Storagebar (Autodesk Fusion 360 design; units mm, degrees)
Autodesk Fusion 360 part; units mm, degrees
sketch "Sketch1" plane through (0, 0, 0) normal (1, 0, 0) x (0, 1, 0)
  circle A0 centre (0, 0) radius 9
  dimension "d1" = 18
  constraint coincident A0.centre origin
  measures "d1" diameter of A0
extrude "Extrude1" add sketch "Sketch1" along normal blind 100 from surface at 5 makes body 1
sketch "Sketch2" plane through (0, 0, 0) normal (1, 0, 0) x (0, 1, 0)
  circle A0 centre (0, 0) radius 9.1
  circle A1 centre (0, 0) radius 12.6
  line L0 (0, 0) -> (-19.9239, 1.7431)
  line L1 (0, 0) -> (20, 0) construction
  line L2 (0, 0) -> (19.9239, 1.7431)
  line L3 (0, 0) -> (20, 0) construction
  circle A2 centre (0, -35) radius 10
  circle A3 centre (0, -35) radius 5
  line L4 (-21.2876, 35.0304) -> (-21.2876, -70)
  line L5 (-13.3685, 9.8483) -> (-9.165, -46.5811)
  line L6 (13.6434, 13.539) -> (8.4962, -55.559)
  circle A4 centre (0, -35) radius 2.5
  circle A5 centre (0, -35) radius 6.5
  line L7 (-35, -35) -> (38.1692, -35)
  line L8 (-10.1926, 14.3296) -> (-4.6115, -60.5935)
  line L9 (10.3108, 15.9153) -> (5.1932, -52.785)
  circle A6 centre (0, 0) radius 2.5
  circle A7 centre (0, 0) radius 5
  dimension "d4" = 18.2
  dimension "d5" = 25.2
  dimension "d8" = 175
  dimension "d9" = 20
  dimension "d10" = 20
  dimension "d11" = 5
  dimension "d14" = 20
  dimension "d15" = 10
  dimension "d16" = 35
  dimension "d17" = 5
  dimension "d18" = 13
  dimension "d27" = 5
  dimension "d28" = 10
  constraint coincident A0.centre A1.centre
  constraint horizontal L1
  constraint horizontal L3
  constraint concentric A2 A3
  constraint vertical L4
  constraint tangent A2 L5
  constraint tangent A1 L5
  constraint tangent A2 L6
  constraint tangent A1 L6
  constraint concentric A2 A4
  constraint concentric A4 A5
  constraint horizontal L7
  constraint coincident A2.centre L7
  constraint tangent A0 L8
  constraint tangent A5 L8
  constraint parallel L6 L9
  constraint tangent A0 L9
  constraint concentric A0 A6
  constraint concentric A0 A7
  measures "d4" diameter of A0
  measures "d5" diameter of A1
  measures "d8" angle of L0 L1
  measures "d9" distance of A0.centre L0.end
  measures "d10" distance of A0.centre L2.end
  measures "d11" angle of L2 L3
  measures "d14" diameter of A2
  measures "d15" diameter of A3
  measures "d16" distance of A0.centre A2.centre
  measures "d17" diameter of A4
  measures "d18" diameter of A5
  measures "d27" diameter of A6
  measures "d28" diameter of A7
extrude "Extrude2" add sketch "Sketch2" along normal blind 5 separate body contours A0 L0 L2 A7 | A0 L2 L9 | A0 L0 L2 A7 | A0 A1 L0 L2 L8 L9 | A0 A1 L8 L9 | A1 L2 L9 | A0 L0 L8 | L0 L2 A6 A7 | L0 L2 A6 A7 | A1 L2 L9 | A1 L0 L8 | A1 A2 L8 L9 | A1 A2 L6 L7 L9 | A1 L0 L8 | L0 L2 A6 | L0 L2 A6 | A1 A2 L5 L7 L8 | A2 A5 L7 L8 L9 | A2 L7 L9 | A2 L7 L8 | A2 L6 L7 | A2 L7 L9 | A5 L7 L9 | A2 L5 L7 | A2 L7 L8 | A5 L7 L8 | A3 A5 L7 | A3 A5 L7 | A2 A5 L8 L9 | A3 A4 L7 | A3 A4 L7 | A4 L7 | A4 L7 makes body 2
extrude "Extrude3" add sketch "Sketch2" along normal blind 15 contours A0 L2 L9 | A0 A1 L8 L9 | A1 L2 L9 | A0 L0 L8 | A1 L0 L8 picked at (11.3282, -1.3785) picked at (-11.3282, -1.3785) bodies 2
extrude "Extrude4" add sketch "Sketch2" along normal blind 8 contours A2 L7 L9 | A2 L7 L8 | A2 A5 L8 L9 picked at (8.7391, -36.1302) picked at (-8.7391, -36.1302) bodies 2
extrude "Extrude5" add sketch "Sketch2" along normal blind 15 contours A1 A2 L6 L7 L9 | A1 A2 L5 L7 L8 | A2 L7 L9 | A2 L7 L8 picked at (8.8106, -34.563) picked at (-8.8106, -34.563) bodies 2
chamfer "Chamfer1" distance 25 distance2 7 1 edges at (15, -8.2729, -35) measured on face at (15, 10.3401, -15.101) on bodies 2
chamfer "Chamfer2" distance 25 distance2 7 1 edges at (15, 8.2729, -35) measured on face at (15, 10.3401, -15.101) on bodies 2
extrude "Extrude6" cut sketch "Sketch2" along normal blind 15 contours L0 L2 A6 | L0 L2 A6 | A4 L7 | A4 L7 bodies 2
chamfer "Chamfer3" distance 4 distance2 1 1 edges at (5, -2.3308, 0.904) measured on face at (5, 6.8967, 3.4743) on bodies 2
chamfer "Chamfer4" distance 4 distance2 1 1 edges at (5, -2.3308, -34.096) measured on face at (5, -4.4677, -26.6434) on bodies 2
